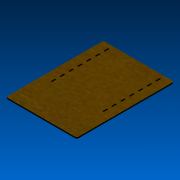
# Autodesk Inventor part: toit
Saved by Autodesk Inventor 2013 SP2 (Build 170200200, 200)
## iProperties
Created: 2015-09-15
Part Number: toit
Material: Generic
Document SubType Name: Modeling
Designer: jeanfrancois
Density: 1 g/cm^3
Author: jeanfrancois
Autodesk Inventor part; units mm, degrees
ref_plane "YZ Plane" through (0, 0, 0) normal (1, 0, 0) x (0, 1, 0)
ref_plane "XZ Plane" through (0, 0, 0) normal (0, 1, 0) x (-1, 0, 0)
ref_plane "XY Plane" through (0, 0, 0) normal (0, 0, 1) x (1, 0, 0)
sketch "Esquisse1" plane through (0, 0, 0) normal (0, 0, 1) x (1, 0, 0)
  line L0 (-91.8695, 89.2103) -> (-91.8695, -122.7897)
  line L1 (-68.8695, 44.1244) -> (-68.8695, 34.1244)
  line L2 (-71.8695, 44.1244) -> (-71.8695, 34.1244)
  line L3 (-71.8695, 24.1244) -> (-71.8695, 14.1244)
  line L4 (-68.8695, 24.1244) -> (-68.8695, 14.1244)
  line L5 (-68.8695, 4.1244) -> (-68.8695, -5.8756)
  line L6 (-71.8695, 4.1244) -> (-71.8695, -5.8756)
  line L7 (-71.8695, 34.1244) -> (-68.8695, 34.1244)
  line L8 (-71.8695, -15.8756) -> (-68.8695, -15.8756)
  line L9 (-71.8695, 24.1244) -> (-68.8695, 24.1244)
  line L10 (-71.8695, 44.1244) -> (-68.8695, 44.1244)
  line L11 (-71.8695, -25.8756) -> (-68.8695, -25.8756)
  line L12 (-71.8695, -5.8756) -> (-68.8695, -5.8756)
  line L13 (-71.8695, 64.1244) -> (-68.8695, 64.1244)
  line L14 (-68.8695, 84.1244) -> (-68.8695, 74.1244)
  line L15 (-71.8695, 84.1244) -> (-71.8695, 74.1244)
  line L16 (-71.8695, 84.1244) -> (-68.8695, 84.1244)
  line L17 (-71.8695, 74.1244) -> (-68.8695, 74.1244)
  line L18 (-68.8695, 64.1244) -> (-68.8695, 54.1244)
  line L19 (-71.8695, 64.1244) -> (-71.8695, 54.1244)
  line L20 (48.1305, -5.8756) -> (45.1305, -5.8756)
  line L21 (-87.8695, 93.2103) -> (64.1305, 93.2103)
  line L22 (68.1305, 89.2103) -> (68.1305, -122.7897)
  line L23 (48.1305, 4.1244) -> (48.1305, -5.8756)
  line L24 (45.1305, 4.1244) -> (45.1305, -5.8756)
  line L25 (48.1305, 4.1244) -> (45.1305, 4.1244)
  line L26 (48.1305, 14.1244) -> (45.1305, 14.1244)
  line L27 (45.1305, 24.1244) -> (45.1305, 14.1244)
  line L28 (48.1305, 24.1244) -> (48.1305, 14.1244)
  line L29 (48.1305, 24.1244) -> (45.1305, 24.1244)
  line L30 (45.1305, 44.1244) -> (45.1305, 34.1244)
  line L31 (48.1305, 44.1244) -> (45.1305, 44.1244)
  line L32 (48.1305, 44.1244) -> (48.1305, 34.1244)
  line L33 (48.1305, 54.1244) -> (45.1305, 54.1244)
  line L34 (45.1305, 64.1244) -> (45.1305, 54.1244)
  line L35 (48.1305, 64.1244) -> (45.1305, 64.1244)
  line L36 (48.1305, 64.1244) -> (48.1305, 54.1244)
  line L37 (48.1305, 74.1244) -> (45.1305, 74.1244)
  line L38 (45.1305, 84.1244) -> (45.1305, 74.1244)
  line L39 (48.1305, 84.1244) -> (45.1305, 84.1244)
  line L40 (48.1305, 84.1244) -> (48.1305, 74.1244)
  line L41 (48.1305, 34.1244) -> (45.1305, 34.1244)
  line L42 (-71.8695, -15.8756) -> (-71.8695, -25.8756)
  line L43 (-68.8695, -15.8756) -> (-68.8695, -25.8756)
  line L44 (-68.8695, -35.8756) -> (-68.8695, -45.8756)
  line L45 (48.1305, -15.8756) -> (45.1305, -15.8756)
  line L46 (45.1305, -15.8756) -> (45.1305, -25.8756)
  line L47 (48.1305, -15.8756) -> (48.1305, -25.8756)
  line L48 (48.1305, -25.8756) -> (45.1305, -25.8756)
  line L49 (48.1305, -35.8756) -> (45.1305, -35.8756)
  line L50 (48.1305, -35.8756) -> (48.1305, -45.8756)
  line L51 (48.1305, -45.8756) -> (45.1305, -45.8756)
  line L52 (-87.8695, -126.7897) -> (64.1305, -126.7897)
  line L53 (-71.8695, -35.8756) -> (-68.8695, -35.8756)
  line L54 (-71.8695, -35.8756) -> (-71.8695, -45.8756)
  line L55 (-71.8695, -45.8756) -> (-68.8695, -45.8756)
  line L56 (45.1305, -35.8756) -> (45.1305, -45.8756)
  line L57 (-71.8695, 14.1244) -> (-68.8695, 14.1244)
  line L58 (-71.8695, 54.1244) -> (-68.8695, 54.1244)
  line L59 (-71.8695, 4.1244) -> (-68.8695, 4.1244)
  arc A0 (-87.8695, 93.2103) -> (-91.8695, 89.2103) centre (-87.8695, 89.2103) ccw
  arc A1 (68.1305, 89.2103) -> (64.1305, 93.2103) centre (64.1305, 89.2103) ccw
  arc A2 (64.1305, -126.7897) -> (68.1305, -122.7897) centre (64.1305, -122.7897) ccw
  arc A3 (-91.8695, -122.7897) -> (-87.8695, -126.7897) centre (-87.8695, -122.7897) ccw
  point P0 (0, 0)
  point P1 (-91.8695, 93.2103)
  point P2 (-91.8695, -126.7897)
  point P3 (68.1305, 93.2103)
  point P4 (68.1305, -126.7897)
  dimension "d3" = 220
  dimension "d5" = 4
  constraints: 120 end point, 8 point on circle, 8 point on line, 8 tangent, 4 centre point, 3 equal radius, 1 horizontal
  measures "d3" distance between parallel lines of L21 L52
  measures "d5" radius of A0
extrude "Extrusion1" add sketch "Esquisse1" along normal blind 3
